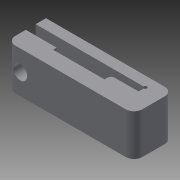
# Autodesk Inventor part: Loop
Saved by Autodesk Inventor 2014 SP1 (Build 180222100, 222)
## iProperties
Created: 2017-02-10
Part Number: Loop
Material: Generic
Document SubType Name: Modeling
Designer: danielsikar
Density: 1 g/cm^3
Appearance: Default
Author: danielsikar
Autodesk Inventor part; units mm, degrees
ref_plane "YZ Plane" through (0, 0, 0) normal (1, 0, 0) x (0, 1, 0)
ref_plane "XZ Plane" through (0, 0, 0) normal (0, 1, 0) x (-1, 0, 0)
ref_plane "XY Plane" through (0, 0, 0) normal (0, 0, 1) x (1, 0, 0)
sketch "Sketch1" plane through (0, 0, 0) normal (0, 0, 1) x (1, 0, 0)
  line L0 (22.0635, 29.031) -> (22.0741, 29.031)
  line L1 (22.0635, 29.031) -> (22.0635, 28.8989)
  arc A0 (22.0635, 28.8989) -> (22.0653, 28.8449) centre (22.893, 28.8989) ccw
  line L2 (22.893, 28.0694) -> (48.1914, 28.0694)
  arc A1 (48.6061, 27.6547) -> (48.1914, 28.0694) centre (48.6061, 28.0694) ccw
  line L3 (48.6061, 27.6547) -> (48.6061, 26.4105)
  line L4 (48.6061, 26.4105) -> (42.7999, 26.4105)
  arc A2 (42.7999, 26.4105) -> (41.9705, 25.581) centre (42.7999, 25.581) ccw
  line L5 (41.9705, 25.581) -> (41.9705, 23.4245)
  line L6 (29.5286, 23.4245) -> (41.9705, 23.4245)
  line L7 (29.5286, 25.6909) -> (29.5286, 23.4245)
  line L8 (22.0635, 25.6909) -> (29.5286, 25.6909)
  line L9 (22.0635, 33.3622) -> (52.8128, 33.3622)
  line L10 (52.8128, 33.3622) -> (52.8128, 19.4198)
  line L11 (52.8128, 19.4198) -> (22.0635, 19.4198)
  line L12 (22.0635, 19.4198) -> (22.0635, 33.3622)
  line L13 (21.7606, 28.8449) -> (22.0653, 28.8449)
  line L14 (56.2668, 28.0694) -> (56.2411, 28.0694)
  line L15 (22.0635, 25.6909) -> (30.348, 25.6909)
  line L16 (42.7999, 26.4105) -> (48.6061, 26.4105)
  line L17 (22.0635, 34.9405) -> (22.0635, 17.9582)
  line L18 (17.0806, 21.0245) -> (52.8128, 21.0245)
  line L19 (48.1914, 28.0694) -> (22.0635, 28.0694)
  line L20 (14.2529, 30.3694) -> (52.8128, 30.3694)
  dimension "d0" = 2.4
  dimension "d2" = 2.3
  constraints: 42 end point, 7 point on circle, 6 point on line, 5 parallel, 4 perpendicular, 3 centre point, 1 horizontal
  measures "d0" distance between parallel lines of L18 L6
  measures "d2" distance between parallel lines of L20 L2
extrude "Extrusion1" add sketch "Sketch1" along normal blind 10 contours L12 L20 L10 L18 L8 L7 L6 L5 A2 L4 L3 A1 L2 L19 A0 L1 | L12 L9 L10 L20 | L10 L11 L12 L18
sketch "Sketch2" plane through (0, 0, 10) normal (0, 0, 1) x (1, 0, 0)
  line L0 (22.0635, 28.0694) -> (48.1914, 28.0694) projected
  line L1 (41.9705, 23.4245) -> (29.5286, 23.4245) projected
  line L2 (22.0635, 25.6909) -> (22.0635, 19.4198) projected
  line L3 (52.8128, 19.4198) -> (52.8128, 33.3622) projected
  line L4 (22.0635, 33.3622) -> (52.8128, 33.3622)
  line L5 (52.8128, 33.3622) -> (52.8128, 30.5694)
  line L6 (52.8128, 30.5694) -> (22.0635, 30.5694)
  line L7 (22.0635, 30.5694) -> (22.0635, 33.3622)
  line L8 (52.8128, 19.4198) -> (22.0635, 19.4198)
  line L9 (22.0635, 19.4198) -> (22.0635, 21.1245)
  line L10 (22.0635, 21.1245) -> (52.8128, 21.1245)
  line L11 (52.8128, 21.1245) -> (52.8128, 19.4198)
  point P0 (0, 0)
  dimension "d5" = 2.5
  dimension "d6" = 2.3
  constraints: 16 end point, 4 parallel, 2 horizontal, 2 perpendicular, 2 point on line
  measures "d5" distance between parallel lines of L6 L0
  measures "d6" distance between parallel lines of L10 L1
extrude "Extrusion2" cut sketch "Sketch2" against normal blind 10
fillet "Fillet1" radius 2 3 edges at (52.8128, 30.5694, 5) (52.8128, 21.1245, 5) (22.0635, 21.1245, 5)
sketch "Sketch3" plane through (22.0635, 30.5694, 10) normal (0, 1, 0) x (1, 0, 0)
  line L0 (0, 0) -> (0, 10) projected
  circle A0 centre (3.2, 5) radius 1.7
  point P0 (-22.0635, 10)
  dimension "d10" = 3.4
  dimension "d11" = 3.2
  constraints: 1 centre point
  measures "d10" diameter of A0
  measures "d11" distance from line of A0.centre L0
extrude "Extrusion3" cut sketch "Sketch3" against normal blind 10
sketch "Sketch4" plane through (29.5286, 23.4245, 0) normal (0, 1, 0) x (1, 0, 0)
  line L0 (0, 0) -> (12.4418, 0) projected
  line L1 (0, 0) -> (0, -10) projected
  line L2 (12.4418, -10) -> (0, -10) projected
  line L3 (12.4418, 0) -> (12.4418, -10) projected
  point P0 (-29.5286, 0)
extrude "Extrusion4" add sketch "Sketch4" along normal blind 1.4
body "Solid1"
